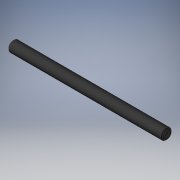
# Autodesk Inventor part: RDOB6-86-WMC3
Saved by Autodesk Inventor 2019 (Build 230136000, 136)
## iProperties
Created: 2022-12-28
Part Number: RDOB6-86-WMC3
Material: Generic
Catalog Web Link: www.cadenas.de
Description: RDOC, RDOB, RDOM, RDSS, RDSSB, RDSSM, RD435S-Rods - Material 1045 Carbon Steel, 1018 Carbon Steel, 4137 Alloy Steel - Outer Diameter Selectable Type
Vendor: MISUMI
Document SubType Name: Modeling
Designer: psAdmin
Manufacturer: MISUMI
Mass: 2.35994 g
Surface Area: 17.6981 cm^2
Volume: 2.35994 cm^3
Density: 1 g/cm^3
Appearance: PSOLRGB-175-175-175
Category: PARTsolutions
Company: MISUMI
Title: RDOB6-86-WMC3
Author: Cadenas PARTsolutions
Comments: Rods - Material 1045 Carbon Steel, 1018 Carbon Steel, 4137 Alloy Steel - Outer Diameter Selectable Type
PSOL_IDENT_0: {$CADENAS_DATA/23d-libs/misumi/metric/22_rods_pipes/rdoc.prj},232 {VTYP=3D},{NB=RDOB6-86-WMC3},{LINA=
PSOL_IDENT_1: RDOB6-86-WMC3},{NN=RDOC, RDOB, RDOM, RDSS, RDSSB, RDSSM, RD435S},{DATE=07.06.2021 02:47:19},{GEOMDAT
PSOL_IDENT_2: E=07.10.2015 00:00:37},{VERSION=},{LINEID=40},{WBVAR=MAT,ST,L,ALT1,MC,WMC},{WBNUMERIC=L,MC,WMC}  {NB=
PSOL_IDENT_3: RDOB6-86-WMC3},{LINA=RDOB6-86-WMC3},{KT=DUMMY},{PN=RDOB6-86-WMC3},{TYPE=RDOB},{MAT=1},{ST=2},{STA='1'
PSOL_IDENT_4: ,'-','2','Black Oxide','3','Electroless Nickel Plating'},{D=6},{DTOL=0/-0.1},{L=86},{LTOL=+/-0.3},{L
PSOL_IDENT_5: 1=[10:500/1]},{C=0.5},{ALT1=2},{ALT1A='3','w/o Tapping','1','with MC (One End Tapping)','2','with WM
PSOL_IDENT_6: C (Both Ends Tapping)'},{MC=0},{MCSA=0},{MCS1=3},{WMC=3},{WMCSA=3},{WMCS1=3},{MMAX=3},{P=0.50},{KDM=
PSOL_IDENT_7: 2.459},{MATA= '1', '1045 Carbon Steel Equivalent', '2', '1018 Carbon Steel' , '3' , 'SCM435' }
NB: RDOB6-86-WMC3
NN: RDOC, RDOB, RDOM, RDSS, RDSSB, RDSSM, RD435S
NT: Rods - Material 1045 Carbon Steel, 1018 Carbon Steel, 4137 Alloy Steel - Outer Diameter Selectable Type
NBSYN: $PN.
LINA: RDOB6-86-WMC3
CATALOG: Misumi
PN: RDOB6-86-WMC3
MAT: 1045 Carbon Steel Equivalent
ST: Black Oxide
D: 6
DTOL: 0/-0.1
L: 86
LTOL: +/-0.3
C: 0.5
ALT1: with WMC (Both Ends Tapping)
MC: 0
WMC: 3
SUPPLIER: MISUMI
ARTICLENO: RDOB6-86-WMC3
BOMINFO: RDOB6-86-WMC3
CREATOR: CADENAS GmbH
Autodesk Inventor part; units mm, degrees
ref_plane "YZ Plane" through (0, 0, 0) normal (1, 0, 0) x (0, 1, 0)
ref_plane "XZ Plane" through (0, 0, 0) normal (0, 1, 0) x (-1, 0, 0)
ref_plane "XY Plane" through (0, 0, 0) normal (0, 0, 1) x (1, 0, 0)
sketch "Sketch_1" plane through (0, 0, 0) normal (0, 0, 1) x (1, 0, 0)
  line L0 (86, 0) -> (0, 0)
  line L1 (0, 0) -> (0, 2.5)
  line L2 (0, 2.5) -> (0.5, 3)
  line L3 (0.5, 3) -> (85.5, 3)
  line L4 (85.5, 3) -> (86, 2.5)
  line L5 (86, 2.5) -> (86, 0)
  line L6 (86, 0) -> (0, 0)
  constraints: 14 end point
revolve "Revolution1" add sketch "Sketch_1" angle 360 about axis through (86, 0, 0) along (1, 0, 0)
sketch "Sketch2" plane through (0, 0, 0) normal (-1, 0, 0) x (0, 0, 1)
  point P0 (0, 0)
hole "Hole1" at (0, 0, 0) direction (1, 0, 0) diameter 2.459 depth 6.7901 tip angle 120 countersink diameter 3 countersink angle 90 thread size "M3x0.5" class "6H" standard "ISO Metric profile"
sketch "Sketch3" plane through (86, 0, 0) normal (1, 0, 0) x (0, 0, -1)
  point P0 (0, 0)
hole "Hole2" at (86, 0, 0) direction (-1, 0, 0) diameter 2.459 depth 6.7601 tip angle 120 countersink diameter 3 countersink angle 90 thread size "M3x0.5" class "6H" standard "ISO Metric profile"
body "Solid1"
